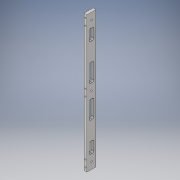
# Autodesk Inventor part: slides
Saved by Autodesk Inventor 2019 (Build 230136000, 136)
## iProperties
Created: 2019-05-04
Part Number: slides
Material: Generic
Document SubType Name: Modeling
Designer: Delta
Density: 1 g/cm^3
Appearance: Default
Author: Delta
Autodesk Inventor part; units mm, degrees
ref_plane "YZ Plane" through (0, 0, 0) normal (1, 0, 0) x (0, 1, 0)
ref_plane "XZ Plane" through (0, 0, 0) normal (0, 1, 0) x (-1, 0, 0)
ref_plane "XY Plane" through (0, 0, 0) normal (0, 0, 1) x (1, 0, 0)
sketch "Sketch1" plane through (0, 0, 0) normal (1, 0, 0) x (0, 1, 0)
  line L0 (0, 0) -> (300, 0)
  line L1 (300, 0) -> (300, 20)
  line L2 (300, 20) -> (0, 20)
  line L3 (0, 20) -> (0, 0)
  dimension "d0" = 300
  dimension "d1" = 20
  constraints: 8 end point, 2 parallel, 1 horizontal, 1 perpendicular
  measures "d0" distance of L1.end L2.end
  measures "d1" distance of L0.end L1.end
extrude "Extrusion1" add sketch "Sketch1" along normal blind 6.35
sketch "Sketch2" plane through (6.35, 0, 0) normal (1, 0, 0) x (0, 0, -1)
  line L0 (0, 300) -> (-20, 300) projected
  line L1 (-20, 300) -> (-20, 0) projected
  line L2 (-20, 0) -> (0, 0) projected
  point P0 (-10, 285)
  point P1 (-10, 150)
  point P2 (-10, 15)
  dimension "d4" = 15
  dimension "d5" = 20
  dimension "d6" = 10
  dimension "d7" = 15
  dimension "d8" = 10
  dimension "d9" = 10
  dimension "d10" = 150
  measures "d4" distance from line of L0 point (-10, 285)
  measures "d5" distance of L0.start L0.end
  measures "d6" distance from line of L1 point (-10, 285)
  measures "d7" distance from line of L2 point (-10, 15)
  measures "d8" distance from line of L1 point (-10, 15)
  measures "d9" distance from line of L1 point (-10, 150)
  measures "d10" distance from line of L0 point (-10, 150)
hole "Hole1" at (6.35, 285, 10) at (6.35, 150, 10) at (6.35, 15, 10) direction (-1, 0, 0) diameter 3.3 end through all
sketch "Sketch5" plane through (6.35, 0, 0) normal (1, 0, 0) x (0, 0, -1)
  line L0 (-15, 270) -> (-5, 270)
  line L1 (-5, 270) -> (-5, 245)
  line L2 (-5, 245) -> (-15, 245)
  line L3 (-15, 245) -> (-15, 270)
  line L4 (-15, 205) -> (-5, 205)
  line L5 (-5, 205) -> (-5, 165)
  line L6 (-5, 165) -> (-15, 165)
  line L7 (-15, 165) -> (-15, 205)
  line L8 (-15, 135) -> (-5, 135)
  line L9 (-5, 135) -> (-5, 95)
  line L10 (-5, 95) -> (-15, 95)
  line L11 (-15, 95) -> (-15, 135)
  line L12 (-15, 55) -> (-5, 55)
  line L13 (-5, 55) -> (-5, 30)
  line L14 (-5, 30) -> (-15, 30)
  line L15 (-15, 30) -> (-15, 55)
  line L16 (0, 0) -> (0, 300) projected
  line L17 (-20, 300) -> (-20, 0) projected
  line L18 (0, 300) -> (-20, 300) projected
  line L19 (-20, 0) -> (0, 0) projected
  dimension "d44" = 5
  dimension "d45" = 5
  dimension "d46" = 30
  dimension "d47" = 30
  dimension "d48" = 55
  dimension "d49" = 95
  dimension "d50" = 135
  dimension "d51" = 55
  dimension "d52" = 95
  dimension "d53" = 135
  constraints: 32 end point, 8 parallel, 6 point on line, 4 horizontal, 4 perpendicular
  measures "d44" distance between parallel lines of L16 L1
  measures "d45" distance between parallel lines of L17 L3
  measures "d46" distance between parallel lines of L18 L0
  measures "d47" distance between parallel lines of L19 L14
  measures "d48" distance between parallel lines of L2 L18
  measures "d49" distance between parallel lines of L18 L4
  measures "d50" distance between parallel lines of L18 L6
  measures "d51" distance between parallel lines of L19 L12
  measures "d52" distance between parallel lines of L10 L19
  measures "d53" distance between parallel lines of L8 L19
extrude "Extrusion2" cut sketch "Sketch5" against normal through all contours L0 L1 L2 L3 | L4 L5 L6 L7 | L8 L9 L10 L11 | L12 L13 L14 L15
fillet "Fillet1" radius 3.175 1 edges at (3.175, 270, 5)
fillet "Fillet2" radius 3.175 1 edges at (3.175, 270, 15)
fillet "Fillet3" radius 3.175 1 edges at (3.175, 245, 5)
fillet "Fillet4" radius 3.175 1 edges at (3.175, 245, 15)
fillet "Fillet5" radius 3.175 1 edges at (3.175, 205, 5)
fillet "Fillet6" radius 3.175 1 edges at (3.175, 205, 15)
fillet "Fillet7" radius 3.175 1 edges at (3.175, 165, 5)
fillet "Fillet8" radius 3.175 1 edges at (3.175, 165, 15)
fillet "Fillet9" radius 3.175 1 edges at (3.175, 95, 5)
fillet "Fillet10" radius 3.175 1 edges at (3.175, 135, 5)
fillet "Fillet11" radius 3.175 1 edges at (3.175, 135, 15)
fillet "Fillet12" radius 3.175 1 edges at (3.175, 95, 15)
fillet "Fillet13" radius 3.175 1 edges at (3.175, 55, 5)
fillet "Fillet14" radius 3.175 1 edges at (3.175, 55, 15)
fillet "Fillet15" radius 3.175 1 edges at (3.175, 30, 15)
fillet "Fillet16" radius 3.175 1 edges at (3.175, 30, 5)
sketch "Sketch7" plane through (0, 0, 0) normal (0, 0, -1) x (-1, 0, 0)
  line L0 (0, 300) -> (-6.35, 300) projected
  line L1 (0, 0) -> (-6.35, 0) projected
  line L2 (-6.35, 0) -> (-6.35, 300) projected
  point P0 (-3.175, 7.5)
  point P1 (-3.175, 22.5)
  point P2 (-3.175, 142.5)
  point P3 (-3.175, 157.5)
  point P4 (-3.175, 277.5)
  point P5 (-3.175, 292.5)
  dimension "d72" = 7.5
  dimension "d73" = 22.5
  dimension "d74" = 142.5
  dimension "d78" = 7.5
  dimension "d79" = 22.5
  dimension "d82" = 142.5
  dimension "d83" = 6.35
  dimension "d84" = 3.175
  dimension "d85" = 3.175
  dimension "d88" = 3.175
  dimension "d89" = 3.175
  dimension "d92" = 3.175
  dimension "d93" = 3.175
  measures "d72" distance from line of L0 point (-3.175, 292.5)
  measures "d73" distance from line of point (-3.175, 277.5) L0
  measures "d74" distance from line of L0 point (-3.175, 157.5)
  measures "d78" distance from line of point (-3.175, 7.5) L1
  measures "d79" distance from line of L1 point (-3.175, 22.5)
  measures "d82" distance from line of L1 point (-3.175, 142.5)
  measures "d83" distance of L0.start L0.end
  measures "d84" distance from line of L2 point (-3.175, 292.5)
  measures "d85" distance from line of L2 point (-3.175, 277.5)
  measures "d88" distance from line of L2 point (-3.175, 157.5)
  measures "d89" distance from line of L2 point (-3.175, 142.5)
  measures "d92" distance from line of L2 point (-3.175, 22.5)
  measures "d93" distance from line of L2 point (-3.175, 7.5)
hole "Hole3" at (3.175, 7.5, 0) at (3.175, 22.5, 0) at (3.175, 142.5, 0) at (3.175, 157.5, 0) at (3.175, 277.5, 0) at (3.175, 292.5, 0) direction (0, 0, 1) diameter 2.6416 end through all thread size "6-32 UNC" class "2B" standard "ANSI Unified Screw Threads"
equation "\"d6\" = 0.5 * d5"
equation "\"d7\" = d4"
equation "\"d8\" = d6"
equation "\"d9\" = d6"
equation "\"d45\" = d44"
equation "\"d47\" = d46"
equation "\"d51\" = d48"
equation "\"d52\" = d49"
equation "\"d53\" = d50"
equation "\"d78\" = d72"
equation "\"d79\" = d73"
equation "\"d82\" = d74"
equation "\"d84\" = 0.5 * d83"
equation "\"d85\" = d84"
equation "\"d88\" = d87"
equation "\"d89\" = d88"
equation "\"d92\" = d91"
equation "\"d93\" = d91"
equation "\"d87\" = d84"
equation "\"d91\" = d89"
body "Solid1"
